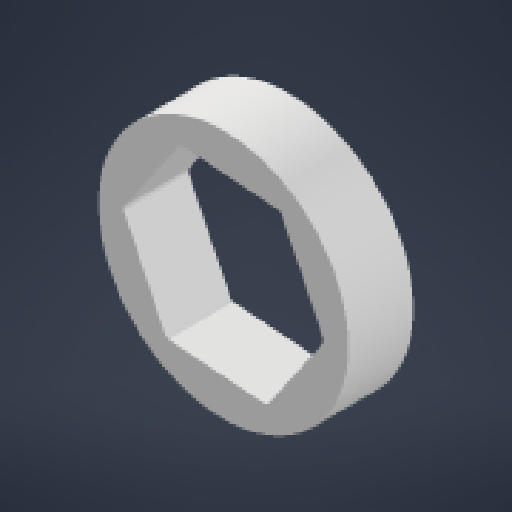
# Autodesk Inventor part: Power_Transmission_Spacer_One
Saved by Autodesk Inventor 2024.2 (Build 282272000, 272)
## iProperties
Created: 2024-03-30
Part Number: Power_Transmission_Spacer_One
Material: Generic
Document SubType Name: Modeling
Designer: warm
Density: 1 g/cm^3
Appearance: Default
Author: warm
Autodesk Inventor part; units mm, degrees
ref_plane "YZ Plane" through (0, 0, 0) normal (1, 0, 0) x (0, 1, 0)
ref_plane "XZ Plane" through (0, 0, 0) normal (0, 1, 0) x (-1, 0, 0)
sketch "Sketch1" plane through (0, 0, 0) normal (0, 0, 1) x (1, 0, 0)
  line L0 (3.9818, -0.3812) -> (1.7924, -3.5759)
  arc A0 (1.6608, -3.6389) -> (1.7924, -3.5759) centre (0, 0) ccw
  line L1 (1.6608, -3.6389) -> (-2.2007, -3.3402)
  arc A1 (-2.321, -3.2577) -> (-2.2007, -3.3402) centre (0, 0) ccw
  line L2 (-2.321, -3.2577) -> (-3.993, 0.2357)
  arc A2 (-3.9818, 0.3812) -> (-3.993, 0.2357) centre (0, 0) ccw
  line L3 (-3.9818, 0.3812) -> (-1.7924, 3.5759)
  arc A3 (-1.6608, 3.6389) -> (-1.7924, 3.5759) centre (0, 0) ccw
  line L4 (-1.6608, 3.6389) -> (2.2007, 3.3402)
  arc A4 (2.321, 3.2577) -> (2.2007, 3.3402) centre (0, 0) ccw
  line L5 (2.321, 3.2577) -> (3.993, -0.2357)
  arc A5 (3.9818, -0.3812) -> (3.993, -0.2357) centre (0, 0) ccw
  circle A6 centre (0, 0) radius 5
  point P0 (0, 0)
  dimension "d0" = 10
  constraints: 12 end point, 12 point on circle, 7 centre point, 1 coincident, 30 other
  measures "d0" diameter of A6
ref_plane "Work Plane1" through (-9.2786, -9.2786, 2.6) normal (0, 0, -1) x (0, 1, 0)
extrude "Extrusion1" add sketch "Sketch1" along normal up to surface (2.6 mm away)
body "Solid1"
